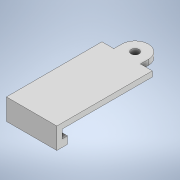
# Autodesk Inventor part: tampa hc12
Saved by Autodesk Inventor 2022 (Build 260153000, 153)
## iProperties
Created: 2022-03-13
Part Number: tampa hc12
Material: Genérico
Document SubType Name: Modeling
Designer: Hanter
Density: 1 g/cm^3
Appearance: Padrão
Author: Hanter
Autodesk Inventor part; units mm, degrees
ref_plane "YZ Plane" through (0, 0, 0) normal (1, 0, 0) x (0, 1, 0)
ref_plane "XZ Plane" through (0, 0, 0) normal (0, 1, 0) x (-1, 0, 0)
ref_plane "XY Plane" through (0, 0, 0) normal (0, 0, 1) x (1, 0, 0)
sketch "Esboço1" plane through (0, 0, 0) normal (1, 0, 0) x (0, 1, 0)
  line L0 (0, 0) -> (-3.2, 0)
  line L1 (-6, 0) -> (-6, 2)
  line L2 (-6, 2) -> (2, 2)
  line L3 (2, 2) -> (2, -42)
  line L4 (2, -42) -> (0, -42)
  line L5 (0, -42) -> (0, 0)
  line L6 (-6, 0) -> (-6, -2)
  line L7 (-6, -2) -> (-3.2, -2)
  line L8 (-3.2, -2) -> (-3.2, 0)
  dimension "d0" = 6
  dimension "d1" = 2
  dimension "d2" = 8
  dimension "d3" = 44
  dimension "d4" = 2
  dimension "d5" = 2.8
  constraints: 18 end point, 7 perpendicular, 1 horizontal, 1 vertical
  measures "d0" distance of L0.start L1.start
  measures "d1" distance of L1.start L1.end
  measures "d2" distance of L1.end L2.end
  measures "d3" distance of L2.end L3.end
  measures "d4" distance of L1.start L6.end
  measures "d5" distance of L6.end L7.end
extrude "Extrusão1" add sketch "Esboço1" along normal blind 19
sketch "Esboço2" plane through (0, 2, 2) normal (0, 1, 0) x (1, 0, 0)
  line L0 (0, 44) -> (19, 44) projected
  line L1 (14.5, 44) -> (14.5, 36)
  line L2 (4.5, 36) -> (4.5, 44)
  line L3 (0, 44) -> (0, 0) projected
  line L4 (4.5, 36) -> (0, 36)
  line L5 (0, 36) -> (0, 44)
  line L6 (0, 44) -> (4.5, 44)
  line L7 (4.5, 44) -> (4.5, 36)
  line L8 (19, 44) -> (19, 0) projected
  line L9 (14.5, 36) -> (19, 36)
  line L10 (19, 36) -> (19, 44)
  line L11 (19, 44) -> (14.5, 44)
  line L12 (14.5, 44) -> (14.5, 36)
  point P0 (0, 2)
  point P1 (0, 36)
  constraints: 20 end point, 5 parallel, 2 horizontal, 2 perpendicular, 1 point on line
extrude "Extrusão2" cut sketch "Esboço2" against normal blind 19
fillet "Arredondamento1" radius 5 2 edges at (14.5, 1, -42) (4.5, 1, -42)
sketch "Esboço3" plane through (0, 2, 2) normal (0, 1, 0) x (1, 0, 0)
  circle A0 centre (9.5, 39) radius 1.5
  line L0 (14.5, 36) -> (14.5, 39) projected
  arc A1 (14.5, 39) -> (4.5, 39) centre (9.5, 39) ccw projected
  point P0 (0, 2)
  dimension "d14" = 3
  dimension "d15" = 5
  dimension "d16" = 0
  constraints: 1 centre point
  measures "d14" diameter of A0
  measures "d15" distance from line of L0 A0.centre
  measures "d16" distance of A1.centre A0.centre
extrude "Extrusão3" cut sketch "Esboço3" against normal blind 19
